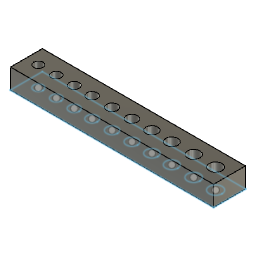
M3 Screw Tester v1 (Autodesk Fusion 360 design; units mm, degrees)
Autodesk Fusion 360 part; units mm, degrees
sketch "Sketch1" plane through (0, 0, 0) normal (0, 0, 1) x (1, 0, 0)
  line L0 (5, 24) -> (56, 24)
  line L1 (56, 24) -> (56, 16)
  line L2 (56, 16) -> (5, 16)
  line L3 (5, 16) -> (5, 24)
  circle A0 centre (8, 20) radius 1.15
  circle A1 centre (12.5, 20) radius 1.2
  circle A2 centre (17, 20) radius 1.25
  circle A3 centre (21.5, 20) radius 1.3
  circle A4 centre (26.5, 20) radius 1.35
  circle A5 centre (31.5, 20) radius 1.4
  circle A6 centre (36.5, 20) radius 1.45
  circle A7 centre (41.5, 20) radius 1.5
  circle A8 centre (47, 20) radius 1.55
  circle A9 centre (52.5, 20) radius 1.6
  dimension "d1" = 51
  dimension "d2" = 8
  dimension "d6" = 2.3
  dimension "d7" = 2.4
  dimension "d8" = 2.5
  dimension "d9" = 2.6
  dimension "d10" = 2.7
  dimension "d11" = 2.8
  dimension "d12" = 2.9
  dimension "d13" = 3
  dimension "d14" = 3.1
  dimension "d15" = 3.2
  constraint horizontal L0
  constraint vertical L1
  constraint horizontal L2
  constraint vertical L3
  measures "d1" distance of L0.start L0.end
  measures "d2" distance of L0.end L1.end
  measures "d6" diameter of A0
  measures "d7" diameter of A1
  measures "d8" diameter of A2
  measures "d9" diameter of A3
  measures "d10" diameter of A4
  measures "d11" diameter of A5
  measures "d12" diameter of A6
  measures "d13" diameter of A7
  measures "d14" diameter of A8
  measures "d15" diameter of A9
extrude "Extrude2" add sketch "Sketch1" along normal blind 5
